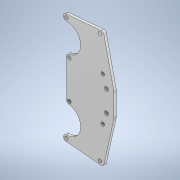
# Autodesk Inventor part: 膝_メインフレーム_1
Saved by Autodesk Inventor 2020 (Build 240168000, 168)
## iProperties
Created: 2021-09-05
Part Number: 膝_メインフレーム_1
Material: アルミニウム 2014-T4
Document SubType Name: Modeling
Designer: masato
Density: 2.8 g/cm^3
Appearance: サテン
Mass: 15.1185 g
Surface Area: 61.8531 cm^2
Volume: 5.39947 cm^3
Author: masato
Autodesk Inventor part; units mm, degrees
ref_plane "YZ Plane" through (0, 0, 0) normal (1, 0, 0) x (0, 1, 0)
ref_plane "XZ Plane" through (0, 0, 0) normal (0, 1, 0) x (-1, 0, 0)
ref_plane "XY Plane" through (0, 0, 0) normal (0, 0, 1) x (1, 0, 0)
sketch "スケッチ1" plane through (0, 0, 0) normal (0, 0, 1) x (1, 0, 0)
  line L0 (-32.2352, 43.3932) -> (10.6011, 47.1409) construction
  line L1 (10.6011, 47.1409) -> (13.3901, 15.2627) construction
  line L2 (13.3901, 15.2627) -> (-29.4462, 11.515) construction
  line L3 (-29.4462, 11.515) -> (-32.2352, 43.3932) construction
  line L4 (-32.2352, 43.3932) -> (13.3901, 15.2627) construction
  line L5 (10.6011, 47.1409) -> (-29.4462, 11.515) construction
  line L6 (-30.8407, 27.4541) -> (11.9956, 31.2018) construction
  line L7 (7.8305, 44.389) -> (-19.0668, 42.0358) construction
  line L8 (-19.0668, 42.0358) -> (-16.7136, 15.1385) construction
  line L9 (-16.7136, 15.1385) -> (10.1837, 17.4917) construction
  line L10 (10.1837, 17.4917) -> (7.8305, 44.389) construction
  line L11 (7.8305, 44.389) -> (-16.7136, 15.1385) construction
  line L12 (-19.0668, 42.0358) -> (10.1837, 17.4917) construction
  circle A0 centre (-18.8864, 28.5) radius 10.5 construction
  circle A1 centre (-19.0668, 42.0358) radius 1.35
  line L13 (-5.6182, 43.2124) -> (-3.265, 16.3151) construction
  circle A2 centre (7.8305, 44.389) radius 1.35
  circle A3 centre (-16.7136, 15.1385) radius 1.35
  circle A4 centre (10.1837, 17.4917) radius 1.35
  arc A5 (-21.4577, 41.8266) -> (-19.0348, 39.636) centre (-19.0668, 42.0358) ccw
  arc A6 (-17.0988, 17.5074) -> (-19.0348, 39.636) centre (-18.8864, 28.5) ccw
  arc A7 (-17.0988, 17.5074) -> (-19.1136, 15.1385) centre (-16.7136, 15.1385) ccw
  line L14 (-21.4577, 41.8266) -> (-21.6756, 44.3171)
  circle A8 centre (13.1136, 8.5) radius 1.55
  circle A9 centre (13.1136, 8.5) radius 6 construction
  circle A10 centre (13.1136, 8.5) radius 4.6 construction
  line L15 (19.1136, 8.5) -> (19.1136, -8.5)
  line L16 (-19.1136, 15.1385) -> (-19.1136, -15.1385)
  line L17 (-19.1136, 0) -> (19.1136, 0) construction
  line L18 (-21.6756, 44.3171) -> (10.6011, 47.1409)
  line L19 (10.6011, 47.1409) -> (18.9683, 9.8123)
  arc A11 (19.1136, 8.5) -> (18.9683, 9.8123) centre (13.1136, 8.5) ccw
  circle A12 centre (-18.8864, -28.5) radius 10.5 construction
  circle A13 centre (-19.0668, -42.0358) radius 1.35
  circle A14 centre (7.8305, -44.389) radius 1.35
  circle A15 centre (-16.7136, -15.1385) radius 1.35
  circle A16 centre (10.1837, -17.4917) radius 1.35
  arc A17 (-19.0348, -39.636) -> (-21.4577, -41.8266) centre (-19.0668, -42.0358) ccw
  arc A18 (-19.0348, -39.636) -> (-17.0988, -17.5074) centre (-18.8864, -28.5) ccw
  arc A19 (-19.1136, -15.1385) -> (-17.0988, -17.5074) centre (-16.7136, -15.1385) ccw
  line L20 (-21.4577, -41.8266) -> (-21.6756, -44.3171)
  circle A20 centre (13.1136, -8.5) radius 1.55
  circle A21 centre (13.1136, -8.5) radius 6 construction
  line L21 (-21.6756, -44.3171) -> (10.6011, -47.1409)
  line L22 (10.6011, -47.1409) -> (18.9683, -9.8123)
  arc A22 (18.9683, -9.8123) -> (19.1136, -8.5) centre (13.1136, -8.5) ccw
  point P0 (0, 0)
  point P1 (-9.4225, 29.328)
  point P2 (-4.4416, 29.7638)
  dimension "d21" = 43
  dimension "d22" = 32
  dimension "d23" = 27
  dimension "d24" = 27
  dimension "d27" = 21
  dimension "d28" = 9.5
  dimension "d29" = 2.7
  dimension "d30" = 2.4
  dimension "d31" = 3.1
  dimension "d34" = 12
  dimension "d39" = 8.5
  dimension "d40" = 9.2
  dimension "d41" = 32
  dimension "d43" = 5
  dimension "d45" = 17
  dimension "d46" = 20
  dimension "d47" = 57
  constraints: 46 end point, 22 centre point, 22 symmetric about line, 18 point on circle, 12 midpoint, 9 coincident, 6 parallel, 5 tangent, 4 perpendicular, 3 point on line, 2 vertical, 18 other
  measures "d21" distance of L1.end L2.end
  measures "d22" distance of L0.end L1.end
  measures "d23" distance of L9.end L8.end
  measures "d24" distance of L8.end L7.end
  measures "d27" diameter of A0
  measures "d28" distance of point (-9.423, 29.328) A0.centre
  measures "d29" diameter of A1
  measures "d30" radius of A5
  measures "d31" diameter of A8
  measures "d34" diameter of A9
  measures "d39" distance from line of L8 point (-9.423, 29.328)
  measures "d40" diameter of A10
  measures "d41" horizontal distance of A8.centre A0.centre
  measures "d43" angle of L17 L2
  measures "d45" distance of A20.centre A8.centre
  measures "d46" vertical distance of A11.centre A0.centre
  measures "d47" distance of A18.centre A0.centre
extrude "押し出し1" add sketch "スケッチ1" along normal blind 2
fillet "フィレット1" radius 2 4 edges at (-21.6756, 44.3171, 1) (-21.6756, -44.3171, 1) (10.6011, -47.1409, 1) (10.6011, 47.1409, 1)
